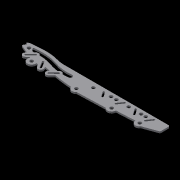
# Autodesk Inventor part: ForearmBaseLeft
Saved by Autodesk Inventor 2015 (Build 190159000, 159)
## iProperties
Created: 2014-10-05
Part Number: ForearmBaseLeft
Material: Generic
Document SubType Name: Modeling
Designer: Val
Density: 1 g/cm^3
Appearance: Default
Mass: 16.0754 g
Surface Area: 143.019 cm^2
Volume: 16.0754 cm^3
Author: Val
Autodesk Inventor part; units mm, degrees
ref_plane "YZ Plane" through (0, 0, 0) normal (1, 0, 0) x (0, 1, 0)
ref_plane "XZ Plane" through (0, 0, 0) normal (0, 1, 0) x (-1, 0, 0)
ref_plane "XY Plane" through (0, 0, 0) normal (0, 0, 1) x (1, 0, 0)
sketch "Base" plane through (0, 0, 0) normal (0, 0, 1) x (1, 0, 0)
  line L0 (-88.2296, 29.6083) -> (-106.7296, 28.2173)
  arc A0 (-106.7296, 28.2173) -> (-111.5, 25.1921) centre (-106.2797, 22.2342) ccw
  line L1 (-111.5, 25.1921) -> (-113.9649, 20.8419)
  arc A1 (-113.9649, 20.8419) -> (-111.808, 14.4812) centre (-110.0497, 18.6235) ccw
  line L2 (-111.808, 14.4812) -> (-98.6963, 8.9156)
  arc A2 (-98.6963, 8.9156) -> (-90.9909, 3.6412) centre (-94.3497, 7) ccw
  line L3 (-90.9909, 3.6412) -> (-90.0412, 4.591)
  arc A3 (-86.4745, -0.307) -> (-90.0412, 4.591) centre (-98.4774, -5.3) ccw
  arc A4 (-86.4745, -0.307) -> (-72.7826, -0.6602) centre (-79.5497, 2.5735) ccw
  arc A5 (-66.25, -1.7001) -> (-72.7826, -0.6602) centre (-71, -10.5) ccw
  arc A6 (-66.25, -1.7001) -> (-57.9832, 2.9682) centre (-62.2, 0.7817) ccw
  arc A7 (-57.9832, 2.9682) -> (-51.2774, 1.3823) centre (11.1884, 280.4773) ccw
  arc A8 (-51.2774, 1.3823) -> (-43.7004, -4.1001) centre (-47, -0.6832) ccw
  line L4 (-43.7004, -4.1001) -> (-40.3291, -0.8445)
  arc A9 (-40.3291, -0.8445) -> (-5.5616, -5.0318) centre (11.1884, 280.4773) ccw
  arc A10 (-59.3435, 26.7816) -> (-88.2296, 29.6083) centre (-81.8939, -54.6538) ccw
  arc A11 (-59.3435, 26.7816) -> (-46, 24.9682) centre (-46, 74.9682) ccw
  arc A12 (-5.5616, -5.0318) -> (5.6654, -4.9146) centre (0, 0) ccw
  line L5 (5.6654, -4.9146) -> (53.6654, -3.2384)
  arc A13 (53.6654, -3.2384) -> (65.7753, -2.6463) centre (59.5047, 1.4682) ccw
  line L6 (65.7753, -2.6463) -> (99.8785, -0.8584)
  arc A14 (99.8785, -0.8584) -> (112.3745, -0.491) centre (106.0047, 3.4682) ccw
  line L7 (112.3745, -0.491) -> (136.3745, 8.2153)
  line L8 (165.7955, 19.8419) -> (164.8009, 23.8311) construction
  arc A15 (165.1662, 18.6599) -> (165.7955, 19.8419) centre (164.8252, 19.6) ccw construction
  line L9 (-46, 24.9682) -> (136.3745, 24.9682)
  arc A16 (164.8009, 23.8311) -> (163.3454, 24.9682) centre (163.3454, 23.4682) ccw construction
  line L10 (136.3745, 24.9682) -> (136.3745, 8.2153)
  line L11 (136.3745, 24.9682) -> (163.3454, 24.9682) construction
  line L12 (136.3745, 8.2153) -> (165.1662, 18.6599) construction
  point P0 (164.5173, 24.9682)
  point P1 (-90.5161, 4.1161)
  dimension "d49" = 1.5
  dimension "d50" = 24
  constraints: 34 point on circle, 26 end point, 17 centre point, 4 horizontal, 3 tangent, 2 point on line, 1 midpoint, 1 vertical, 26 other
  measures "d49" radius of A16
  measures "d50" distance from line of L10 L7.start
extrude "BaseFeature" add sketch "Base" along normal blind 3
sketch "ExternalAssemblyGeometry" plane through (0, 0, 3) normal (0, 0, 1) x (1, 0, 0)
  circle A0 centre (72.3941, 17.9682) radius 2.4585
  circle A1 centre (51.0047, 17.9682) radius 2.4585
  circle A2 centre (42.0047, 17.9682) radius 2.4585
  line L0 (112.4005, 21.3286) -> (106.0987, 12.3286)
  arc A3 (106.0987, 12.3286) -> (108.5561, 10.6079) centre (107.3274, 11.4682) ccw
  line L1 (108.5561, 10.6079) -> (114.858, 19.6079)
  arc A4 (114.858, 19.6079) -> (112.4005, 21.3286) centre (113.6293, 20.4682) ccw
  line L2 (89.4685, 12.3286) -> (83.1667, 21.3286)
  arc A5 (83.1667, 21.3286) -> (80.7092, 19.6079) centre (81.9379, 20.4682) ccw
  line L3 (80.7092, 19.6079) -> (87.0111, 10.6079)
  arc A6 (87.0111, 10.6079) -> (89.4685, 12.3286) centre (88.2398, 11.4682) ccw
  circle A7 centre (72.3941, 17.9682) radius 2.4585
  line L4 (57.7772, 10.6079) -> (64.0791, 19.6079)
  arc A8 (64.0791, 19.6079) -> (61.6216, 21.3286) centre (62.8503, 20.4682) ccw
  line L5 (61.6216, 21.3286) -> (55.3198, 12.3286)
  arc A9 (55.3198, 12.3286) -> (57.7772, 10.6079) centre (56.5485, 11.4682) ccw
  circle A10 centre (134.0047, 23.9682) radius 1.2295
  circle A11 centre (158.0047, 23.9682) radius 1.2295
  circle A12 centre (72.3941, 17.9682) radius 2.4585
  circle A13 centre (93.7836, 17.9682) radius 2.4585
  circle A14 centre (101.7836, 17.9682) radius 2.4585
  line L6 (-39.0502, 9.079) -> (-48.042, 0.3958)
  arc A15 (-36.9663, 6.921) -> (-39.0502, 9.079) centre (-38.0083, 8) ccw
  line L7 (-45.958, -1.7622) -> (-36.9663, 6.921)
  arc A16 (-48.042, 0.3958) -> (-45.958, -1.7622) centre (-47, -0.6832) ccw
  arc A17 (-63.479, -0.002) -> (-60.921, 1.5655) centre (-62.2, 0.7817) ccw
  line L8 (-60.921, 1.5655) -> (-67.4523, 12.2235)
  line L9 (-70.0102, 10.656) -> (-63.479, -0.002)
  arc A18 (-67.4523, 12.2235) -> (-70.0102, 10.656) centre (-68.7312, 11.4398) ccw
  line L10 (-93.289, 5.9393) -> (-84.4502, 14.7782)
  arc A19 (-84.4502, 14.7782) -> (-86.5715, 16.8995) centre (-85.5109, 15.8388) ccw
  line L11 (-86.5715, 16.8995) -> (-95.4104, 8.0607)
  arc A20 (-95.4104, 8.0607) -> (-93.289, 5.9393) centre (-94.3497, 7) ccw
  circle A21 centre (13.3989, 15.9682) radius 2.4585
  line L12 (35.5355, 11.5467) -> (30.0865, 19.3286)
  arc A22 (33.078, 9.8259) -> (35.5355, 11.5467) centre (34.3067, 10.6863) ccw
  arc A23 (30.0865, 19.3286) -> (27.629, 17.6079) centre (28.8578, 18.4682) ccw
  line L13 (27.629, 17.6079) -> (33.078, 9.8259)
  line L14 (-95.4104, 8.0607) -> (-86.5715, 16.8995)
  arc A24 (-95.4104, 8.0607) -> (-93.289, 5.9393) centre (-94.3497, 7) ccw
  line L15 (-84.4502, 14.7782) -> (-93.289, 5.9393)
  arc A25 (-84.4502, 14.7782) -> (-86.5715, 16.8995) centre (-85.5109, 15.8388) ccw
  arc A26 (-67.4523, 12.2235) -> (-70.0102, 10.656) centre (-68.7312, 11.4398) ccw
  line L16 (-63.479, -0.002) -> (-70.0102, 10.656)
  line L17 (-67.4523, 12.2235) -> (-60.921, 1.5655)
  arc A27 (-63.479, -0.002) -> (-60.921, 1.5655) centre (-62.2, 0.7817) ccw
  line L18 (-48.042, 0.3958) -> (-39.0502, 9.079)
  arc A28 (-48.042, 0.3958) -> (-45.958, -1.7622) centre (-47, -0.6832) ccw
  line L19 (-36.9663, 6.921) -> (-45.958, -1.7622)
  arc A29 (-36.9663, 6.921) -> (-39.0502, 9.079) centre (-38.0083, 8) ccw
  line L20 (33.078, 9.8259) -> (27.629, 17.6079)
  arc A30 (30.0865, 19.3286) -> (27.629, 17.6079) centre (28.8578, 18.4682) ccw
  line L21 (30.0865, 19.3286) -> (35.5355, 11.5467)
  arc A31 (55.3198, 12.3286) -> (57.7772, 10.6079) centre (56.5485, 11.4682) ccw
  line L22 (64.0791, 19.6079) -> (57.7772, 10.6079)
  line L23 (55.3198, 12.3286) -> (61.6216, 21.3286)
  arc A32 (64.0791, 19.6079) -> (61.6216, 21.3286) centre (62.8503, 20.4682) ccw
  arc A33 (83.1667, 21.3286) -> (80.7092, 19.6079) centre (81.9379, 20.4682) ccw
  line L24 (87.0111, 10.6079) -> (80.7092, 19.6079)
  line L25 (83.1667, 21.3286) -> (89.4685, 12.3286)
  arc A34 (87.0111, 10.6079) -> (89.4685, 12.3286) centre (88.2398, 11.4682) ccw
  line L26 (106.0987, 12.3286) -> (112.4005, 21.3286)
  arc A35 (114.858, 19.6079) -> (112.4005, 21.3286) centre (113.6293, 20.4682) ccw
  line L27 (114.858, 19.6079) -> (108.5561, 10.6079)
  arc A36 (106.0987, 12.3286) -> (108.5561, 10.6079) centre (107.3274, 11.4682) ccw
  arc A37 (-102.0167, 23.4581) -> (-101.0827, 16.5207) centre (-101.5497, 19.9894) ccw construction
  spline S0 degree 3 poles (-20.9034, 11.8689) (-20.699, 12.2669) (-20.5753, 12.705) (-20.4895, 13.5682) (-20.5334, 14.0463) (-20.8057, 14.9369) (-21.0336, 15.3499) (-21.5235, 15.9479) (-21.7901, 16.193) (-22.0935, 16.3926) knots 0.402356 0.402356 0.402356 0.402356 0.529128 0.529128 0.66478 0.66478 0.800432 0.800432 0.906058 0.906058 0.906058 0.906058
  arc A38 (-55.7151, 20.4123) -> (-24.4179, 16.9452) centre (-32.5, 86.9804) ccw
  arc A39 (-22.0935, 16.3926) -> (-24.4179, 16.9452) centre (-24.0166, 13.4682) ccw
  arc A40 (-55.7151, 20.4123) -> (-82.5497, 24.8435) centre (-81.8939, -54.6538) ccw
  arc A41 (-82.5497, 24.8435) -> (-98.0321, 23.9424) centre (-81.267, -130.6512) ccw
  spline S1 degree 3 poles (-102.0167, 23.4581) (-102.2026, 23.4331) (-102.3877, 23.3929) (-103.0138, 23.2025) (-103.4291, 22.9741) (-104.1043, 22.4214) (-104.4106, 22.059) (-104.8528, 21.2372) (-104.9886, 20.7776) (-105.0359, 20.302) (-105.0388, 20.268) (-105.0412, 20.2339) knots 0 0 0 0 0.116037 0.116037 0.403242 0.403242 0.690649 0.690649 0.978056 0.978056 1 1 1 1 construction
  arc A42 (-90.5061, 17.5611) -> (-101.0827, 16.5207) centre (-81.267, -130.6512) ccw construction
  arc A43 (-58.0202, 13.8027) -> (-81.2043, 17.8429) centre (-81.8939, -54.6538) ccw
  arc A44 (-58.0202, 13.8027) -> (-42.6253, 10.1446) centre (-32.5, 86.9804) ccw
  arc A45 (-33.4969, 9.4868) -> (-23.6154, 9.9913) centre (-32.5, 86.9804) ccw
  arc A46 (-58.0202, 13.8027) -> (-81.2043, 17.8429) centre (-81.8939, -54.6538) ccw
  arc A47 (-81.2043, 17.8429) -> (-88.8696, 19.1976) centre (-85.5109, 15.8388) ccw
  arc A48 (-33.4969, 9.4868) -> (-41.3079, 11.4169) centre (-38.0083, 8) ccw
  line L28 (-41.3079, 11.4169) -> (-42.6253, 10.1446)
  arc A49 (-23.6154, 9.9913) -> (-24.4179, 16.9452) centre (-24.0166, 13.4682) ccw
  line L29 (-88.8696, 19.1976) -> (-90.5061, 17.5611)
  arc A50 (-98.0321, 23.9424) -> (-90.5061, 17.5611) centre (-90.9491, 24.6673) ccw
  point P0 (0, 0)
  constraints: 82 point on circle, 60 end point, 51 centre point, 1 equal radius, 1 tangent, 139 other
sketch "Rails" plane through (0, 0, 3) normal (0, 0, 1) x (1, 0, 0)
  arc A0 (-98.0321, 23.9424) -> (-90.5061, 17.5611) centre (-90.9491, 24.6673) ccw projected
  arc A1 (-82.5497, 24.8435) -> (-98.0321, 23.9424) centre (-81.267, -130.6512) ccw projected
  line L0 (-88.8696, 19.1976) -> (-90.5061, 17.5611) projected
  arc A2 (-81.2043, 17.8429) -> (-88.8696, 19.1976) centre (-85.5109, 15.8388) ccw projected
  arc A3 (-55.7151, 20.4123) -> (-82.5497, 24.8435) centre (-81.8939, -54.6538) ccw projected
  arc A4 (-58.0202, 13.8027) -> (-81.2043, 17.8429) centre (-81.8939, -54.6538) ccw projected
  arc A5 (-55.7151, 20.4123) -> (-24.4179, 16.9452) centre (-32.5, 86.9804) ccw projected
  arc A6 (-58.0202, 13.8027) -> (-42.6253, 10.1446) centre (-32.5, 86.9804) ccw projected
  line L1 (-41.3079, 11.4169) -> (-42.6253, 10.1446) projected
  arc A7 (-33.4969, 9.4868) -> (-41.3079, 11.4169) centre (-38.0083, 8) ccw projected
  arc A8 (-33.4969, 9.4868) -> (-23.6154, 9.9913) centre (-32.5, 86.9804) ccw projected
  arc A9 (-23.6154, 9.9913) -> (-24.4179, 16.9452) centre (-24.0166, 13.4682) ccw projected
  line L2 (-86.5715, 16.8995) -> (-95.4104, 8.0607) projected
  arc A10 (-84.4502, 14.7782) -> (-86.5715, 16.8995) centre (-85.5109, 15.8388) ccw projected
  line L3 (-93.289, 5.9393) -> (-84.4502, 14.7782) projected
  arc A11 (-95.4104, 8.0607) -> (-93.289, 5.9393) centre (-94.3497, 7) ccw projected
  arc A12 (-67.4523, 12.2235) -> (-70.0102, 10.656) centre (-68.7312, 11.4398) ccw projected
  line L4 (-70.0102, 10.656) -> (-63.479, -0.002) projected
  line L5 (-60.921, 1.5655) -> (-67.4523, 12.2235) projected
  arc A13 (-63.479, -0.002) -> (-60.921, 1.5655) centre (-62.2, 0.7817) ccw projected
  arc A14 (-48.042, 0.3958) -> (-45.958, -1.7622) centre (-47, -0.6832) ccw projected
  line L6 (-39.0502, 9.079) -> (-48.042, 0.3958) projected
  line L7 (-45.958, -1.7622) -> (-36.9663, 6.921) projected
  arc A15 (-36.9663, 6.921) -> (-39.0502, 9.079) centre (-38.0083, 8) ccw projected
  arc A16 (30.0865, 19.3286) -> (27.629, 17.6079) centre (28.8578, 18.4682) ccw projected
  line L8 (27.629, 17.6079) -> (33.078, 9.8259) projected
  line L9 (35.5355, 11.5467) -> (30.0865, 19.3286) projected
  arc A17 (33.078, 9.8259) -> (35.5355, 11.5467) centre (34.3067, 10.6863) ccw projected
  arc A18 (55.3198, 12.3286) -> (57.7772, 10.6079) centre (56.5485, 11.4682) ccw projected
  line L10 (61.6216, 21.3286) -> (55.3198, 12.3286) projected
  line L11 (57.7772, 10.6079) -> (64.0791, 19.6079) projected
  arc A19 (64.0791, 19.6079) -> (61.6216, 21.3286) centre (62.8503, 20.4682) ccw projected
  arc A20 (83.1667, 21.3286) -> (80.7092, 19.6079) centre (81.9379, 20.4682) ccw projected
  line L12 (80.7092, 19.6079) -> (87.0111, 10.6079) projected
  line L13 (83.1667, 21.3286) -> (89.4685, 12.3286) projected
  arc A21 (87.0111, 10.6079) -> (89.4685, 12.3286) centre (88.2398, 11.4682) ccw projected
  arc A22 (106.0987, 12.3286) -> (108.5561, 10.6079) centre (107.3274, 11.4682) ccw projected
  line L14 (112.4005, 21.3286) -> (106.0987, 12.3286) projected
  line L15 (108.5561, 10.6079) -> (114.858, 19.6079) projected
  arc A23 (114.858, 19.6079) -> (112.4005, 21.3286) centre (113.6293, 20.4682) ccw projected
  point P0 (0, 0)
extrude "RailsFeature" cut sketch "Rails" against normal through all
sketch "BaseHoles" plane through (0, 0, 0) normal (0, 0, -1) x (-1, 0, 0)
  arc A0 (-112.3745, -0.491) -> (-99.8785, -0.8584) centre (-106.0047, 3.4682) ccw projected
  arc A1 (-65.7753, -2.6463) -> (-53.6654, -3.2384) centre (-59.5047, 1.4682) ccw projected
  arc A2 (72.7826, -0.6602) -> (86.4745, -0.307) centre (79.5497, 2.5735) ccw projected
  point P0 (0, 0)
hole "BaseHolesFeature" at (106.0047, 3.4682, 0) at (59.5047, 1.4682, 0) at (0, 0, 0) at (-79.5497, 2.5735, 0) direction (0, 0, 1) diameter 6 end through all
hole "TopHolesFeature" at (13.3989, 15.9682, 3) at (42.0047, 17.9682, 3) at (51.0047, 17.9682, 3) at (72.3941, 17.9682, 3) at (93.7836, 17.9682, 3) at (101.7836, 17.9682, 3) direction (0, 0, -1) diameter 6 end through all
hole "CableConnectorHoleFeature" at (-101.5497, 19.9894, 3) direction (0, 0, -1) diameter 6 end through all
fillet "LipFilletFeature" radius 1 1 edges at (-98.0321, 23.9424, 1.5)
sketch "BottomCut" plane through (0, 0, 0) normal (0, 0, -1) x (-1, 0, 0)
  circle A0 centre (0, 0) radius 7.5 construction
  line L0 (34.7086, 4.5831) -> (43.7004, -4.1001) construction
  arc A1 (43.7004, -4.1001) -> (50.2996, 2.7336) centre (47, -0.6832) ccw construction
  line L1 (50.2996, 2.7336) -> (41.3079, 11.4169) construction
  arc A2 (58.15, 3.2636) -> (66.25, -1.7001) centre (62.2, 0.7817) ccw construction
  line L2 (64.6812, 13.9216) -> (58.15, 3.2636) construction
  line L3 (66.25, -1.7001) -> (72.7813, 8.9579) construction
  circle A3 centre (79.5497, 2.5735) radius 7.5 construction
  line L4 (82.1521, 12.4801) -> (90.9909, 3.6412) construction
  line L5 (111.808, 14.4812) -> (98.6963, 8.9156) construction
  arc A4 (90.9909, 3.6412) -> (97.7085, 10.3588) centre (94.3497, 7) ccw construction
  line L6 (97.7085, 10.3588) -> (88.8696, 19.1976) construction
  arc A5 (5.5616, -5.0318) -> (7.2497, -1.9214) centre (0, 0) ccw
  line L7 (40.3291, -0.8445) -> (37.667, 1.7263)
  arc A6 (7.2497, -1.9214) -> (37.667, 1.7263) centre (-11.1884, 280.4773) ccw
  arc A7 (5.5616, -5.0318) -> (40.3291, -0.8445) centre (-11.1884, 280.4773) ccw construction
  arc A8 (51.2774, 1.3822) -> (50.2996, 2.7336) centre (47, -0.6832) ccw
  arc A9 (58.15, 3.2636) -> (57.9832, 2.9682) centre (62.2, 0.7817) ccw
  line L8 (58.15, 3.2636) -> (59.5592, 5.5632)
  line L9 (50.2996, 2.7336) -> (49.242, 3.755)
  line L10 (49.242, 3.755) -> (59.5592, 5.5632)
  line L11 (37.667, 1.7263) -> (49.242, 3.755) construction
  spline S0 degree 3 poles (66.25, -1.7001) (66.5643, -1.5305) (66.8904, -1.3763) (68.4306, -0.7484) (69.754, -0.5) (71.5837, -0.5) (72.185, -0.5519) (72.7826, -0.6602) knots 6.889606 6.889606 6.889606 6.889606 6.993358 6.993358 7.367164 7.367164 7.542287 7.542287 7.542287 7.542287 construction
  spline S1 degree 3 poles (86.4745, -0.307) (86.4805, -0.2926) (86.4865, -0.2782) (86.7701, 0.3967) (87.1364, 1.1052) (88.0113, 2.4528) (88.5202, 3.0914) (89.3475, 3.9657) (89.6837, 4.286) (90.0412, 4.591) knots 8.690868 8.690868 8.690868 8.690868 8.695828 8.695828 8.923068 8.923068 9.150308 9.150308 9.288316 9.288316 9.288316 9.288316 construction
  arc A10 (72.7826, -0.6602) -> (66.25, -1.7001) centre (71, -10.5) ccw
  line L12 (66.25, -1.7001) -> (69.2537, 3.2014)
  arc A11 (72.1358, 3.7065) -> (72.7826, -0.6602) centre (79.5497, 2.5735) ccw
  line L13 (69.2537, 3.2014) -> (72.1358, 3.7065)
  arc A12 (90.0412, 4.591) -> (86.4745, -0.307) centre (98.4774, -5.3) ccw
  arc A13 (86.4745, -0.307) -> (86.0711, 6.2777) centre (79.5497, 2.5735) ccw
  line L14 (90.0412, 4.591) -> (87.2128, 7.4194)
  line L15 (86.0711, 6.2777) -> (87.2128, 7.4194)
  arc A14 (98.6963, 8.9156) -> (97.7085, 10.3588) centre (94.3497, 7) ccw
  line L16 (98.6963, 8.9156) -> (111.808, 14.4812)
  arc A15 (111.808, 14.4812) -> (113.9649, 20.8419) centre (110.0497, 18.6235) ccw
  line L17 (97.7085, 10.3588) -> (96.728, 11.3392)
  line L18 (113.9649, 20.8419) -> (111.5, 25.1921)
  line L19 (111.5, 25.1921) -> (113.9649, 20.8419) construction
  line L20 (96.728, 11.3392) -> (110.6358, 17.2427)
  arc A16 (110.6358, 17.2427) -> (111.3548, 19.3629) centre (110.0497, 18.6235) ccw
  line L21 (111.3548, 19.3629) -> (108.8899, 23.7131)
  line L22 (108.8899, 23.7131) -> (111.5, 25.1921)
  arc A17 (5.5616, -5.0318) -> (40.3291, -0.8445) centre (-11.1884, 280.4773) ccw
  line L23 (56.8375, 1.0987) -> (57.9832, 2.9682)
  line L24 (51.2774, 1.3822) -> (51.8375, 0.2224)
  arc A18 (43.7004, -4.1001) -> (51.2774, 1.3823) centre (47, -0.6832) ccw projected
  line L25 (56.8375, 1.0987) -> (51.8375, 0.2224)
  dimension "d39" = 3
  dimension "d40" = 4
  dimension "d41" = 4
  dimension "d42" = 3
  dimension "d52" = 5
  constraints: 36 end point, 27 point on circle, 12 centre point, 12 concentric, 6 point on line, 5 parallel, 5 tangent, 2 collinear, 2 perpendicular, 3 other
  measures "d39" radial gap between concentric circles of A7 A6
  measures "d40" distance between parallel lines of L10 L13
  measures "d41" distance of L14.end L14.start
  measures "d42" distance between parallel lines of L5 L20
  measures "d52" horizontal distance of L23.start L24.end
extrude "BottomCutFeature" cut sketch "BottomCut" against normal through all
sketch "SecondaryBottomCut" plane through (0, 0, 0) normal (0, 0, -1) x (-1, 0, 0)
  arc A0 (-112.3745, -0.491) -> (-99.8785, -0.8584) centre (-106.0047, 3.4682) ccw construction
  arc A1 (-65.7753, -2.6463) -> (-53.6654, -3.2384) centre (-59.5047, 1.4682) ccw construction
  line L0 (-65.7753, -2.6463) -> (-99.8785, -0.8584) construction
  circle A2 centre (-106.0047, 3.4682) radius 7.5 construction
  circle A3 centre (-59.5047, 1.4682) radius 7.5 construction
  line L1 (-99.8785, -0.8584) -> (-65.7753, -2.6463)
  arc A4 (-99.8785, -0.8584) -> (-98.515, 3.0756) centre (-106.0047, 3.4682) ccw
  arc A5 (-67.0046, 1.4237) -> (-65.7753, -2.6463) centre (-59.5047, 1.4682) ccw
  line L2 (-98.515, 3.0756) -> (-67.0046, 1.4237)
  line L3 (-65.7753, -2.6463) -> (-99.8785, -0.8584) projected
  dimension "d46" = 4
  constraints: 8 point on circle, 4 centre point, 4 concentric, 4 end point, 2 coincident, 1 parallel
  measures "d46" distance between parallel lines of L0 L2
extrude "SecondaryBottomCutFeature" cut sketch "SecondaryBottomCut" against normal through all
fillet "BaseFilletsFeature" radius 2 2 edges at (136.3745, 8.2153, 1.5) (136.3745, 24.9682, 1.5)
